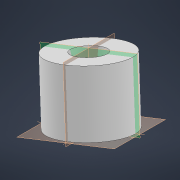
# Autodesk Inventor part: sauce bottle holder
Saved by Autodesk Inventor 2021 (Build 250183000, 183)
## iProperties
Created: 2020-10-21
Part Number: sauce bottle holder
Material: Generic
Document SubType Name: Modeling
Designer: brand
Density: 1 g/cm^3
Appearance: Default
Author: brand
Autodesk Inventor part; units mm, degrees
sketch "Sketch1" plane through (0, 0, 0) normal (0, 0, 1) x (1, 0, 0)
  circle A0 centre (0, 0) radius 25
  dimension "d0" = 50
  constraints: 1 centre point, 1 coincident
  measures "d0" diameter of A0
extrude "Extrusion1" add sketch "Sketch1" along normal blind 40
sketch "Sketch4" plane through (0, 0, 0) normal (0, 1, 0) x (-1, 0, 0)
  line L0 (25, 40) -> (-25, 40) projected
  line L1 (0, 40) -> (-10.5, 40)
  line L2 (-10.5, 40) -> (-3.5769, 10)
  line L3 (-3.5769, 10) -> (0, 10)
  line L4 (25, 0) -> (-25, 0) projected
  line L5 (0, 10) -> (0, 40.9001)
  line L6 (31.0819, 14) -> (-35.1776, 14) construction
  line L7 (0, -8.18) -> (0, 49.0801) construction
  point P0 (0, 0)
  dimension "d10" = 10.5
  dimension "d11" = 26
  dimension "d12" = 4
  constraints: 10 end point, 1 collinear, 1 horizontal, 1 midpoint, 1 parallel, 1 perpendicular, 1 point on line
  measures "d10" distance of L1.start L1.end
  measures "d11" distance between parallel lines of L0 L6
  measures "d12" distance between parallel lines of L3 L6
revolve "Revolution1" cut sketch "Sketch4" angle 360 about axis through (0, 0, -10) along (0, 0, 1)
body "Solid1"
